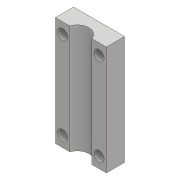
# Autodesk Inventor part: Suspension_Clamp_Cunha
Saved by Autodesk Inventor 2018 (Build 220112000, 112)
## iProperties
Created: 2021-04-28
Part Number: Suspension_Clamp_Cunha
Material: Generic
Document SubType Name: Modeling
Designer: l01767
Density: 1 g/cm^3
Appearance: Default
Author: l01767
Autodesk Inventor part; units mm, degrees
ref_plane "YZ Plane" through (0, 0, 0) normal (1, 0, 0) x (0, 1, 0)
ref_plane "XZ Plane" through (0, 0, 0) normal (0, 1, 0) x (-1, 0, 0)
ref_plane "XY Plane" through (0, 0, 0) normal (0, 0, 1) x (1, 0, 0)
sketch "Sketch1" plane through (0, 0, 0) normal (0, 0, 1) x (1, 0, 0)
  arc A0 (15.1987, 5) -> (-15.1987, 5) centre (0, 0) ccw
  line L0 (-15.1987, 5) -> (-35, 5)
  line L1 (-35, 5) -> (-35, 30)
  line L2 (-35, 30) -> (35, 30)
  line L3 (35, 30) -> (35, 5)
  line L4 (35, 5) -> (15.1987, 5)
  line L5 (0, 0) -> (0, 30)
  dimension "d0" = 32
  dimension "d1" = 70
  dimension "d2" = 5
  dimension "d3" = 19.8013
  dimension "d4" = 25
  constraints: 12 end point, 3 perpendicular, 2 point on circle, 2 point on line, 1 centre point, 1 coincident, 1 horizontal, 1 midpoint, 1 vertical
  measures "d0" diameter of A0
  measures "d1" distance of L1.end L2.end
  measures "d2" distance from line of point (0, 0) L4
  measures "d3" distance of L0.start L0.end
  measures "d4" distance between parallel lines of L0 L2
extrude "Extrusion1" add sketch "Sketch1" along normal mid plane 150
sketch "Sketch2" plane through (-35, 30, 75) normal (0, 1, 0) x (1, 0, 0)
  line L0 (0, 150) -> (70, 150) construction
  line L1 (0, 150) -> (0, 0) construction
  line L2 (35, 75) -> (70, 75)
  line L3 (35, 75) -> (35, 150)
  point P0 (10, 135)
  point P1 (60, 135)
  point P2 (10, 15)
  point P3 (60, 15)
  dimension "d7" = 15
  dimension "d8" = 10
  constraints: 4 end point, 3 symmetric about line, 1 horizontal, 1 midpoint
  measures "d7" distance from line of L0 point (10, 135)
  measures "d8" distance from line of L1 point (10, 135)
hole "Hole1" at (-25, 30, -60) at (25, 30, -60) at (-25, 30, 60) at (25, 30, 60) direction (0, -1, 0) diameter 14 end through all
body "Solid1"
